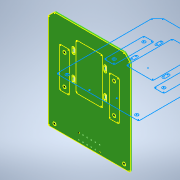
# Autodesk Inventor part: PCB
Saved by Autodesk Inventor 2021 (Build 250183000, 183)
## iProperties
Created: 2020-09-13
Part Number: PCB
Material: Generic
Document SubType Name: Modeling
Designer: Viktor
Density: 1 g/cm^3
Appearance: Default
Author: Viktor
Autodesk Inventor part; units mm, degrees
ref_plane "YZ Plane" through (0, 0, 0) normal (1, 0, 0) x (0, 1, 0)
ref_plane "XZ Plane" through (0, 0, 0) normal (0, 1, 0) x (-1, 0, 0)
ref_plane "XY Plane" through (0, 0, 0) normal (0, 0, 1) x (1, 0, 0)
sketch "Sketch1" plane through (0, 0, 0) normal (0, 0, 1) x (1, 0, 0)
  line L0 (-41.275, -50.8) -> (41.275, -50.8)
  line L1 (41.275, -50.8) -> (41.275, 50.8)
  line L2 (41.275, 50.8) -> (-41.275, 50.8)
  line L3 (-41.275, 50.8) -> (-41.275, -50.8)
  line L4 (-41.275, -50.8) -> (41.275, 50.8) construction
  line L5 (41.275, -50.8) -> (-41.275, 50.8) construction
  circle A0 centre (-35, -46.39) radius 1.6
  circle A1 centre (35, -46.39) radius 1.6
  point P0 (0, 0)
  dimension "d0" = 82.55
  dimension "d1" = 101.6
  dimension "d2" = 3.2
  dimension "d3" = 3.2
  dimension "d5" = 35
  dimension "d6" = 35
  dimension "d7" = 4.41
  dimension "d8" = 4.41
  constraints: 12 end point, 2 centre point, 2 midpoint, 2 parallel, 1 horizontal, 1 perpendicular
  measures "d0" distance of L1.end L2.end
  measures "d1" distance of L0.end L1.end
  measures "d2" diameter of A0
  measures "d3" diameter of A1
  measures "d5" horizontal distance of A1.centre point (0, 0)
  measures "d6" horizontal distance of point (0, 0) A0.centre
  measures "d7" distance from line of L0 A0.centre
  measures "d8" distance from line of L0 A1.centre
extrude "Extrusion1" add sketch "Sketch1" along normal blind 1.6
chamfer "Chamfer1" distance 6 angle 45 1 edges at (41.275, 50.8, 0.8) measured on face at (41.275, -16.9333, 0.5333)
chamfer "Chamfer2" distance 6 angle 45 1 edges at (-41.275, 50.8, 0.8) measured on face at (-41.275, 16.9333, 0.5333)
sketch "Sketch2" plane through (0, 0, 1.6) normal (0, 0, 1) x (1, 0, 0)
  circle A0 centre (-10.48, -42) radius 0.52
  line L0 (-41.275, -50.8) -> (41.275, -50.8) projected
  line L1 (-41.275, 44.8) -> (-41.275, -50.8) projected
  point P0 (0, 0)
  dimension "d17" = 1.04
  dimension "d18" = 10.48
  dimension "d19" = 8.8
  constraints: 1 centre point
  measures "d17" diameter of A0
  measures "d18" horizontal distance of point (0, 0) A0.centre
  measures "d19" distance from line of L0 A0.centre
extrude "Extrusion2" cut sketch "Sketch2" against normal through all
pattern_linear "Rectangular Pattern1" count 6 spacing 4.19 along (1, 0, 0) count 2 spacing 6.35 along (0, -1, 0) of "Extrusion2"
sketch "Sketch3" plane through (0, 0, 1.6) normal (0, 0, 1) x (1, 0, 0)
  circle A0 centre (-25, 20.8) radius 1.6
  circle A1 centre (-25, -9.2) radius 1.6
  line L0 (0, -71.12) -> (0, 71.12) projected
  line L1 (35.275, 50.8) -> (-35.275, 50.8) projected
  circle A2 centre (25, 20.8) radius 1.6
  circle A3 centre (25, -9.2) radius 1.6
  point P0 (0, 0)
  dimension "d28" = 25
  dimension "d29" = 25
  dimension "d30" = 30
  dimension "d31" = 3.2
  dimension "d32" = 3.2
  dimension "d33" = 30
  constraints: 4 centre point, 2 symmetric about line, 2 other
  measures "d28" horizontal distance of point (0, 0) A1.centre
  measures "d29" horizontal distance of point (0, 0) A0.centre
  measures "d30" distance of A1.centre A0.centre
  measures "d31" diameter of A0
  measures "d32" diameter of A1
  measures "d33" distance from line of L1 A0.centre
extrude "Extrusion3" cut sketch "Sketch3" against normal through all
sketch "Sketch4" plane through (0, 0, 1.6) normal (0, 0, 1) x (1, 0, 0)
  line L0 (-16, 0) -> (-16, 4) construction
  line L1 (-14.5, 0) -> (-14.5, 4)
  line L2 (-17.5, 4) -> (-17.5, 0)
  arc A0 (-17.5, 0) -> (-14.5, 0) centre (-16, 0) ccw
  arc A1 (-14.5, 4) -> (-17.5, 4) centre (-16, 4) ccw
  line L3 (-16, 25) -> (-16, 29) construction
  line L4 (-14.5, 25) -> (-14.5, 29)
  line L5 (-17.5, 29) -> (-17.5, 25)
  arc A2 (-17.5, 25) -> (-14.5, 25) centre (-16, 25) ccw
  arc A3 (-14.5, 29) -> (-17.5, 29) centre (-16, 29) ccw
  line L6 (-57.785, 0) -> (57.785, 0) construction
  line L7 (0, 71.12) -> (0, -71.12) projected
  line L8 (16, 0) -> (16, 4) construction
  line L9 (14.5, 0) -> (14.5, 4)
  line L10 (17.5, 4) -> (17.5, 0)
  arc A4 (14.5, 0) -> (17.5, 0) centre (16, 0) ccw
  arc A5 (17.5, 4) -> (14.5, 4) centre (16, 4) ccw
  line L11 (16, 25) -> (16, 29) construction
  line L12 (14.5, 25) -> (14.5, 29)
  line L13 (17.5, 29) -> (17.5, 25)
  arc A6 (14.5, 25) -> (17.5, 25) centre (16, 25) ccw
  arc A7 (17.5, 29) -> (14.5, 29) centre (16, 29) ccw
  line L14 (13.3, -8.625) -> (-13.3, -8.625)
  line L15 (-13.3, -8.625) -> (-13.3, 37.625)
  line L16 (-13.3, 37.625) -> (13.3, 37.625)
  line L17 (13.3, 37.625) -> (13.3, -8.625)
  line L18 (13.3, -8.625) -> (-13.3, 37.625) construction
  line L19 (-13.3, -8.625) -> (13.3, 37.625) construction
  point P0 (0, 0)
  point P1 (-16, 2)
  point P2 (-16, 27)
  point P3 (16, 2)
  point P4 (16, 27)
  point P5 (0, 14.5)
  dimension "d36" = 4
  dimension "d37" = 4
  dimension "d38" = 3
  dimension "d39" = 3
  dimension "d40" = 16
  dimension "d41" = 25
  dimension "d45" = 26.6
  dimension "d46" = 46.25
  dimension "d47" = 12.5
  dimension "d48" = 2
  constraints: 44 end point, 16 point on circle, 14 symmetric about line, 8 centre point, 8 tangent, 5 point on line, 4 midpoint, 4 parallel, 1 horizontal, 1 perpendicular, 1 vertical, 4 other
  measures "d36" distance of L2.start L2.end
  measures "d37" distance of L5.start L5.end
  measures "d38" distance between parallel lines of L2 L1
  measures "d39" distance between parallel lines of L5 L4
  measures "d40" horizontal distance of point (0, 0) point (-16, 2)
  measures "d41" distance of point (-16, 27) point (-16, 2)
  measures "d45" distance of L15.end L16.end
  measures "d46" distance of L14.end L15.end
  measures "d47" vertical distance of point (0, 14.5) point (-16, 2)
  measures "d48" distance from line of L6 point (-16, 2)
extrude "Extrusion4" cut sketch "Sketch4" against normal blind 1.6 contours A0 L2 A1 L1 | A2 L5 A3 L4 | L9 A5 L10 A4 | L12 A7 L13 A6
fillet "Fillet1" radius 1 6 edges at (41.275, -50.8, 0.8) (41.275, 44.8, 0.8) (35.275, 50.8, 0.8) (-35.275, 50.8, 0.8) (-41.275, 44.8, 0.8) (-41.275, -50.8, 0.8)
sketch "RCU_PCB_OUTLINE" plane through (0, 0, 1.6) normal (0, 0, 1) x (1, 0, 0)
  circle A0 centre (-25, 20.8) radius 1.6 projected
  circle A1 centre (25, 20.8) radius 1.6 projected
  circle A2 centre (-25, -9.2) radius 1.6 projected
  circle A3 centre (25, -9.2) radius 1.6 projected
  circle A4 centre (10.47, -48.35) radius 0.52 projected
  circle A5 centre (-10.48, -42) radius 0.52 projected
  circle A6 centre (-35, -46.39) radius 1.6 projected
  circle A7 centre (35, -46.39) radius 1.6 projected
  line L0 (-30, -13.2) -> (-30, 24.8) projected
  line L1 (-30, -13.2) -> (-30, 24.8) projected
  arc A8 (-30, -13.2) -> (-29, -14.2) centre (-29, -13.2) ccw projected
  arc A9 (-29, 25.8) -> (-30, 24.8) centre (-29, 24.8) ccw projected
  arc A10 (-30, -13.2) -> (-29, -14.2) centre (-29, -13.2) ccw projected
  line L2 (-21, -14.2) -> (-29, -14.2) projected
  arc A11 (-21, -14.2) -> (-20, -13.2) centre (-21, -13.2) ccw projected
  line L3 (-20, 24.8) -> (-20, -13.2) projected
  arc A12 (-20, 24.8) -> (-21, 25.8) centre (-21, 24.8) ccw projected
  line L4 (-29, 25.8) -> (-21, 25.8) projected
  arc A13 (-29, 25.8) -> (-30, 24.8) centre (-29, 24.8) ccw projected
  arc A14 (12.3, -8.625) -> (13.3, -7.625) centre (12.3, -7.625) ccw projected
  line L5 (-12.3, -8.625) -> (12.3, -8.625) projected
  arc A15 (-13.3, -7.625) -> (-12.3, -8.625) centre (-12.3, -7.625) ccw projected
  line L6 (-13.3, 36.625) -> (-13.3, -7.625) projected
  arc A16 (-12.3, 37.625) -> (-13.3, 36.625) centre (-12.3, 36.625) ccw projected
  line L7 (12.3, 37.625) -> (-12.3, 37.625) projected
  arc A17 (13.3, 36.625) -> (12.3, 37.625) centre (12.3, 36.625) ccw projected
  line L8 (13.3, -7.625) -> (13.3, 36.625) projected
  line L9 (29, -14.2) -> (21, -14.2) projected
  arc A18 (20, -13.2) -> (21, -14.2) centre (21, -13.2) ccw projected
  line L10 (20, -13.2) -> (20, 24.8) projected
  arc A19 (21, 25.8) -> (20, 24.8) centre (21, 24.8) ccw projected
  line L11 (21, 25.8) -> (29, 25.8) projected
  arc A20 (30, 24.8) -> (29, 25.8) centre (29, 24.8) ccw projected
  line L12 (30, 24.8) -> (30, -13.2) projected
  arc A21 (29, -14.2) -> (30, -13.2) centre (29, -13.2) ccw projected
  line L13 (29, -14.2) -> (21, -14.2) projected
  arc A22 (14.5, 0) -> (17.5, 0) centre (16, 0) ccw projected
  line L14 (17.5, 4) -> (17.5, 0) projected
  arc A23 (17.5, 4) -> (14.5, 4) centre (16, 4) ccw projected
  line L15 (14.5, 0) -> (14.5, 4) projected
  arc A24 (-17.5, 0) -> (-14.5, 0) centre (-16, 0) ccw projected
  line L16 (-14.5, 4) -> (-14.5, 0) projected
  arc A25 (-14.5, 4) -> (-17.5, 4) centre (-16, 4) ccw projected
  line L17 (-17.5, 0) -> (-17.5, 4) projected
  arc A26 (-17.5, 25) -> (-14.5, 25) centre (-16, 25) ccw projected
  line L18 (-14.5, 29) -> (-14.5, 25) projected
  arc A27 (-14.5, 29) -> (-17.5, 29) centre (-16, 29) ccw projected
  line L19 (-17.5, 25) -> (-17.5, 29) projected
  arc A28 (14.5, 25) -> (17.5, 25) centre (16, 25) ccw projected
  line L20 (17.5, 29) -> (17.5, 25) projected
  arc A29 (17.5, 29) -> (14.5, 29) centre (16, 29) ccw projected
  line L21 (14.5, 25) -> (14.5, 29) projected
  line L22 (41.275, -49.8) -> (41.275, 44.3858) projected
  arc A30 (40.275, -50.8) -> (41.275, -49.8) centre (40.275, -49.8) ccw projected
  line L23 (-40.275, -50.8) -> (40.275, -50.8) projected
  arc A31 (-41.275, -49.8) -> (-40.275, -50.8) centre (-40.275, -49.8) ccw projected
  line L24 (-41.275, 44.3858) -> (-41.275, -49.8) projected
  arc A32 (-40.9821, 45.0929) -> (-41.275, 44.3858) centre (-40.275, 44.3858) ccw projected
  line L25 (-40.9821, 45.0929) -> (-35.5679, 50.5071) projected
  arc A33 (-34.8608, 50.8) -> (-35.5679, 50.5071) centre (-34.8608, 49.8) ccw projected
  line L26 (34.8608, 50.8) -> (-34.8608, 50.8) projected
  arc A34 (35.5679, 50.5071) -> (34.8608, 50.8) centre (34.8608, 49.8) ccw projected
  line L27 (35.5679, 50.5071) -> (40.9821, 45.0929) projected
  arc A35 (41.275, 44.3858) -> (40.9821, 45.0929) centre (40.275, 44.3858) ccw projected
  point P0 (0, 0)
  constraints: 8 centre point
equation "\"d6\" = d5"
equation "\"d8\" = d7"
equation "\"d29\" = d28"
equation "\"d32\" = d31"
equation "\"d37\" = d36"
equation "\"d39\" = d38"
equation "\"d47\" = 0.5 * d41"
body "Solid1"
